Autodesk Fusion 360 part; units mm, degrees
note: some values were not read from the file. Chosen so that the rebuilt part matches the saved one: which face or edge a step refers to.
(part 2 of 3)
sketch "Sketch3" plane through (0, 40, 0) normal (0, 1, 0) x (-1, 0, 0)
  line L0 (-7.2987, -37.3386) -> (-8.9484, -42.0586)
  line L1 (-8.9484, -42.0586) -> (-18.3884, -38.7592)
  line L2 (-18.3884, -38.7592) -> (-16.655, -33.7998)
  line L3 (-16.655, -33.7998) -> (-15.239, -34.2947)
  line L4 (-15.239, -34.2947) -> (-15.0741, -33.8227)
  line L5 (-15.0741, -33.8227) -> (-16.514, -33.2432)
  arc A0 (-16.514, -33.2432) -> (-17.1415, -33.4711) centre (-16.7007, -33.7071) ccw
  line L6 (-17.1415, -33.4711) -> (-19.6803, -38.2133)
  line L7 (-19.6803, -38.2133) -> (-21.5, -37.2391)
  line L8 (-21.5, -37.2391) -> (-18.9559, -32.8326)
  arc A1 (-18.9559, -32.8326) -> (-19.1397, -32.0918) centre (-19.4322, -32.5576) ccw
  line L9 (-19.1397, -32.0918) -> (-20.474, -31.254)
  line L10 (-20.474, -31.254) -> (-20.7904, -31.6411)
  line L11 (-20.7904, -31.6411) -> (-19.6291, -32.5905)
  line L12 (-19.6291, -32.5905) -> (-22.7936, -36.4616)
  line L13 (-22.7936, -36.4616) -> (-30.5359, -30.1325)
  line L14 (-30.5359, -30.1325) -> (-27.2108, -26.0651)
  line L15 (-27.2108, -26.0651) -> (-26.0495, -27.0145)
  line L16 (-26.0495, -27.0145) -> (-25.733, -26.6273)
  line L17 (-25.733, -26.6273) -> (-26.888, -25.5903)
  arc A2 (-26.888, -25.5903) -> (-27.5555, -25.5898) centre (-27.222, -25.9623) ccw
  line L18 (-27.5555, -25.5898) -> (-31.5631, -29.1777)
  line L19 (-31.5631, -29.1777) -> (-32.9399, -27.6399)
  line L20 (-32.9399, -27.6399) -> (-29.0421, -24.3692)
  arc A3 (-29.0421, -24.3692) -> (-28.9615, -23.6103) centre (-29.3957, -23.9479) ccw
  line L21 (-28.9615, -23.6103) -> (-29.9287, -22.3667)
  line L22 (-29.9287, -22.3667) -> (-30.3585, -22.6222)
  line L23 (-30.3585, -22.6222) -> (-29.5919, -23.9115)
  line L24 (-29.5919, -23.9115) -> (-33.8896, -26.4669)
  line L25 (-33.8896, -26.4669) -> (-39.0003, -17.8714)
  line L26 (-39.0003, -17.8714) -> (-34.4846, -15.1865)
  line L27 (-34.4846, -15.1865) -> (-33.718, -16.4758)
  line L28 (-33.718, -16.4758) -> (-33.2882, -16.2203)
  line L29 (-33.2882, -16.2203) -> (-34.0188, -14.8508)
  arc A4 (-34.0188, -14.8508) -> (-34.6459, -14.622) centre (-34.46, -15.0861) ccw
  line L30 (-34.6459, -14.622) -> (-39.639, -16.6229)
  line L31 (-39.639, -16.6229) -> (-40.4068, -14.7069)
  line L32 (-40.4068, -14.7069) -> (-35.6255, -12.9666)
  arc A5 (-35.6255, -12.9666) -> (-35.2901, -12.281) centre (-35.8136, -12.4498) ccw
  line L33 (-35.2901, -12.281) -> (-35.7737, -10.7816)
  line L34 (-35.7737, -10.7816) -> (-36.2649, -10.8747)
  line L35 (-36.2649, -10.8747) -> (-35.9855, -12.3485)
  line L36 (-35.9855, -12.3485) -> (-40.898, -13.2798)
  line L37 (-40.898, -13.2798) -> (-42.7607, -3.4548)
  line L38 (-42.7607, -3.4548) -> (-37.599, -2.4762)
  line L39 (-37.599, -2.4762) -> (-37.3196, -3.95)
  line L40 (-37.3196, -3.95) -> (-36.8284, -3.8568)
  line L41 (-36.8284, -3.8568) -> (-37.0465, -2.3201)
  arc A6 (-37.0465, -2.3201) -> (-37.5576, -1.8906) centre (-37.5415, -2.3903) ccw
  line L42 (-37.5576, -1.8906) -> (-42.9338, -2.063)
  line L43 (-42.9338, -2.063) -> (-43, 0)
  line L44 (-43, 0) -> (-37.9118, 0)
  arc A7 (-37.9118, 0) -> (-37.3622, 0.5296) centre (-37.9118, 0.55) ccw
  line L45 (-37.3622, 0.5296) -> (-37.3038, 2.1039)
  line L46 (-37.3038, 2.1039) -> (-37.7972, 2.1844)
  line L47 (-37.7972, 2.1844) -> (-38.0387, 0.704)
  line L48 (-38.0387, 0.704) -> (-42.9735, 1.509)
  line L49 (-42.9735, 1.509) -> (-41.3635, 11.3786)
  line L50 (-41.3635, 11.3786) -> (-36.1784, 10.5327)
  line L51 (-36.1784, 10.5327) -> (-36.4199, 9.0523)
  line L52 (-36.4199, 9.0523) -> (-35.9265, 8.9718)
  line L53 (-35.9265, 8.9718) -> (-35.6058, 10.4905)
  arc A8 (-35.6058, 10.4905) -> (-35.9392, 11.0689) centre (-36.095, 10.5938) ccw
  line L54 (-35.9392, 11.0689) -> (-36.4082, 11.2228)
  line L55 (-41.0502, 12.7456) -> (-40.4068, 14.7069)
  line L56 (-40.4068, 14.7069) -> (-35.6255, 12.9666)
  arc A9 (-35.6255, 12.9666) -> (-34.9278, 13.2763) centre (-35.4373, 13.4834) ccw
  line L57 (-34.9278, 13.2763) -> (-34.3345, 14.7357)
  line L58 (-34.3345, 14.7357) -> (-34.7707, 14.9801)
  line L59 (-34.7707, 14.9801) -> (-35.5039, 13.6716)
  line L60 (-35.5039, 13.6716) -> (-39.8658, 16.1158)
  line L61 (-39.8658, 16.1158) -> (-34.9773, 24.8395)
  line L62 (-34.9773, 24.8395) -> (-30.3942, 22.2713)
  line L63 (-30.3942, 22.2713) -> (-31.1275, 20.9627)
  line L64 (-31.1275, 20.9627) -> (-30.6913, 20.7183)
  line L65 (-30.6913, 20.7183) -> (-29.8706, 22.0358)
  arc A10 (-29.8706, 22.0358) -> (-29.986, 22.6933) centre (-30.2949, 22.3001) ccw
  line L66 (-29.986, 22.6933) -> (-34.2153, 26.0169)
  line L67 (-34.2153, 26.0169) -> (-32.9399, 27.6399)
  line L68 (-32.9399, 27.6399) -> (-29.0421, 24.3692)
  arc A11 (-29.0421, 24.3692) -> (-28.2807, 24.4217) centre (-28.6886, 24.7906) ccw
  line L69 (-28.2807, 24.4217) -> (-27.2239, 25.5901)
  line L70 (-27.2239, 25.5901) -> (-27.5502, 25.969)
  line L71 (-27.5502, 25.969) -> (-28.6868, 24.9901)
  line L72 (-28.6868, 24.9901) -> (-31.9496, 28.7788)
  line L73 (-31.9496, 28.7788) -> (-24.3723, 35.3044)
  line L74 (-24.3723, 35.3044) -> (-20.944, 31.3236)
  line L75 (-20.944, 31.3236) -> (-22.0806, 30.3448)
  line L76 (-22.0806, 30.3448) -> (-21.7543, 29.9659)
  line L77 (-21.7543, 29.9659) -> (-20.5325, 30.9232)
  arc A12 (-20.5325, 30.9232) -> (-20.4161, 31.5805) centre (-20.8408, 31.3168) ccw
  line L78 (-20.4161, 31.5805) -> (-23.2536, 36.1503)
  line L79 (-23.2536, 36.1503) -> (-21.5, 37.2391)
  line L80 (-21.5, 37.2391) -> (-18.9559, 32.8326)
  arc A13 (-18.9559, 32.8326) -> (-18.2224, 32.6214) centre (-18.4796, 33.1076) ccw
  line L81 (-18.2224, 32.6214) -> (-16.8298, 33.358)
  line L82 (-16.8298, 33.358) -> (-17.0068, 33.8256)
  line L83 (-17.0068, 33.8256) -> (-18.4097, 33.2945)
  line L84 (-18.4097, 33.2945) -> (-20.1799, 37.9707)
  line L85 (-20.1799, 37.9707) -> (-10.8276, 41.5111)
  line L86 (-10.8276, 41.5111) -> (-8.9676, 36.5978)
  line L87 (-8.9676, 36.5978) -> (-10.3705, 36.0667)
  line L88 (-10.3705, 36.0667) -> (-10.1934, 35.5991)
  line L89 (-10.1934, 35.5991) -> (-8.7179, 36.0808)
  arc A14 (-8.7179, 36.0808) -> (-8.3837, 36.6587) centre (-8.873, 36.5561) ccw
  line L90 (-8.3837, 36.6587) -> (-9.4871, 41.9233)
  line L91 (-9.4871, 41.9233) -> (-7.4669, 42.3467)
  line L92 (-7.4669, 42.3467) -> (-6.5833, 37.3358)
  arc A15 (-6.5833, 37.3358) -> (-5.9663, 36.8865) centre (-6.0417, 37.4314) ccw
  line L93 (-5.9663, 36.8865) -> (-4.4057, 37.1024)
  line L94 (-4.4057, 37.1024) -> (-4.4122, 37.6023)
  line L95 (-4.4122, 37.6023) -> (-5.912, 37.5831)
  line L96 (-5.912, 37.5831) -> (-5.9762, 42.5827)
  line L97 (-5.9762, 42.5827) -> (4.023, 42.711)
  line L98 (4.023, 42.711) -> (4.0904, 37.4578)
  line L99 (4.0904, 37.4578) -> (2.5905, 37.4386)
  line L100 (2.5905, 37.4386) -> (2.5969, 36.9386)
  line L101 (2.5969, 36.9386) -> (4.1482, 36.8865)
  arc A16 (4.1482, 36.8865) -> (4.6599, 37.3153) centre (4.165, 37.3863) ccw
  line L102 (4.6599, 37.3153) -> (5.4237, 42.6398)
  line L103 (5.4237, 42.6398) -> (7.4669, 42.3467)
  line L104 (7.4669, 42.3467) -> (6.5833, 37.3358)
  arc A17 (6.5833, 37.3358) -> (7.0094, 36.7026) centre (7.125, 37.2403) ccw
  line L105 (7.0094, 36.7026) -> (8.5497, 36.3717)
  line L106 (8.5497, 36.3717) -> (8.7147, 36.8437)
  line L107 (8.7147, 36.8437) -> (7.2987, 37.3386)
  line L108 (7.2987, 37.3386) -> (8.9484, 42.0586)
  line L109 (8.9484, 42.0586) -> (18.3884, 38.7592)
  line L110 (18.3884, 38.7592) -> (16.655, 33.7998)
  line L111 (16.655, 33.7998) -> (15.239, 34.2947)
  line L112 (15.239, 34.2947) -> (15.0741, 33.8227)
  line L113 (15.0741, 33.8227) -> (16.514, 33.2432)
  arc A18 (16.514, 33.2432) -> (17.1415, 33.4711) centre (16.7007, 33.7071) ccw
  line L114 (17.1415, 33.4711) -> (19.6803, 38.2133)
  line L115 (19.6803, 38.2133) -> (21.5, 37.2391)
  line L116 (21.5, 37.2391) -> (18.9559, 32.8326)
  arc A19 (18.9559, 32.8326) -> (19.1397, 32.0918) centre (19.4322, 32.5576) ccw
  line L117 (19.1397, 32.0918) -> (20.474, 31.254)
  line L118 (20.474, 31.254) -> (20.7904, 31.6411)
  line L119 (20.7904, 31.6411) -> (19.6291, 32.5905)
  line L120 (19.6291, 32.5905) -> (22.7936, 36.4616)
  line L121 (22.7936, 36.4616) -> (30.5359, 30.1325)
  line L122 (30.5359, 30.1325) -> (27.2108, 26.0651)
  line L123 (27.2108, 26.0651) -> (26.0495, 27.0145)
  line L124 (26.0495, 27.0145) -> (25.733, 26.6273)
  line L125 (25.733, 26.6273) -> (26.888, 25.5903)
  arc A20 (26.888, 25.5903) -> (27.5555, 25.5898) centre (27.222, 25.9623) ccw
  line L126 (27.5555, 25.5898) -> (31.5631, 29.1777)
  line L127 (31.5631, 29.1777) -> (32.9399, 27.6399)
  line L128 (32.9399, 27.6399) -> (29.0421, 24.3692)
  arc A21 (29.0421, 24.3692) -> (28.9615, 23.6103) centre (29.3957, 23.9479) ccw
  line L129 (28.9615, 23.6103) -> (29.9287, 22.3667)
  line L130 (29.9287, 22.3667) -> (30.3585, 22.6222)
  line L131 (30.3585, 22.6222) -> (29.5919, 23.9115)
  line L132 (29.5919, 23.9115) -> (33.8896, 26.4669)
  line L133 (33.8896, 26.4669) -> (39.0003, 17.8714)
  line L134 (39.0003, 17.8714) -> (34.4846, 15.1865)
  line L135 (34.4846, 15.1865) -> (33.718, 16.4758)
  line L136 (33.718, 16.4758) -> (33.2882, 16.2203)
  line L137 (33.2882, 16.2203) -> (34.0188, 14.8508)
  arc A22 (34.0188, 14.8508) -> (34.6459, 14.622) centre (34.46, 15.0861) ccw
  line L138 (34.6459, 14.622) -> (39.639, 16.6229)
  line L139 (39.639, 16.6229) -> (40.4068, 14.7069)
  line L140 (40.4068, 14.7069) -> (35.6255, 12.9666)
  arc A23 (35.6255, 12.9666) -> (35.2901, 12.281) centre (35.8136, 12.4498) ccw
  line L141 (35.2901, 12.281) -> (35.7737, 10.7816)
  line L142 (35.7737, 10.7816) -> (36.2649, 10.8747)
  line L143 (36.2649, 10.8747) -> (35.9855, 12.3485)
  line L144 (35.9855, 12.3485) -> (40.898, 13.2798)
  line L145 (40.898, 13.2798) -> (42.7607, 3.4548)
  line L146 (42.7607, 3.4548) -> (37.599, 2.4762)
  line L147 (37.599, 2.4762) -> (37.3196, 3.95)
  line L148 (37.3196, 3.95) -> (36.8284, 3.8568)
  line L149 (36.8284, 3.8568) -> (37.0465, 2.3201)
  arc A24 (37.0465, 2.3201) -> (37.5576, 1.8906) centre (37.5415, 2.3903) ccw
  line L150 (37.5576, 1.8906) -> (42.9338, 2.063)
  line L151 (42.9338, 2.063) -> (43, 0)
  line L152 (43, 0) -> (37.9118, 0)
  arc A25 (37.9118, 0) -> (37.3622, -0.5296) centre (37.9118, -0.55) ccw
  line L153 (37.3622, -0.5296) -> (37.3038, -2.1039)
  line L154 (37.3038, -2.1039) -> (37.7972, -2.1844)
  line L155 (37.7972, -2.1844) -> (38.0387, -0.704)
  line L156 (38.0387, -0.704) -> (42.9735, -1.509)
  line L157 (42.9735, -1.509) -> (41.3635, -11.3786)
  line L158 (41.3635, -11.3786) -> (36.1784, -10.5327)
  line L159 (36.1784, -10.5327) -> (36.4199, -9.0523)
  line L160 (36.4199, -9.0523) -> (35.9265, -8.9718)
  line L161 (35.9265, -8.9718) -> (35.6058, -10.4905)
  arc A26 (35.6058, -10.4905) -> (35.9392, -11.0689) centre (36.095, -10.5938) ccw
  line L162 (35.9392, -11.0689) -> (41.0502, -12.7456)
  line L163 (41.0502, -12.7456) -> (40.4068, -14.7069)
  line L164 (40.4068, -14.7069) -> (35.6255, -12.9666)
  arc A27 (35.6255, -12.9666) -> (34.9278, -13.2763) centre (35.4373, -13.4834) ccw
  line L165 (34.9278, -13.2763) -> (34.3345, -14.7357)
  line L166 (34.3345, -14.7357) -> (34.7707, -14.9801)
  line L167 (34.7707, -14.9801) -> (35.5039, -13.6716)
  line L168 (35.5039, -13.6716) -> (39.8658, -16.1158)
  line L169 (39.8658, -16.1158) -> (34.9773, -24.8395)
  line L170 (34.9773, -24.8395) -> (30.3942, -22.2713)
  line L171 (30.3942, -22.2713) -> (31.1275, -20.9627)
  line L172 (31.1275, -20.9627) -> (30.6913, -20.7183)
  line L173 (30.6913, -20.7183) -> (29.8706, -22.0358)
  arc A28 (29.8706, -22.0358) -> (29.986, -22.6933) centre (30.2949, -22.3001) ccw
  line L174 (29.986, -22.6933) -> (34.2153, -26.0169)
  line L175 (34.2153, -26.0169) -> (32.9399, -27.6399)
  line L176 (32.9399, -27.6399) -> (29.0421, -24.3692)
  arc A29 (29.0421, -24.3692) -> (28.2807, -24.4217) centre (28.6886, -24.7906) ccw
  line L177 (28.2807, -24.4217) -> (27.2239, -25.5901)
  line L178 (27.2239, -25.5901) -> (27.5502, -25.969)
  line L179 (27.5502, -25.969) -> (28.6868, -24.9901)
  line L180 (28.6868, -24.9901) -> (31.9496, -28.7788)
  line L181 (31.9496, -28.7788) -> (24.3723, -35.3044)
  line L182 (24.3723, -35.3044) -> (20.944, -31.3236)
  line L183 (20.944, -31.3236) -> (22.0806, -30.3448)
  line L184 (22.0806, -30.3448) -> (21.7543, -29.9659)
  line L185 (21.7543, -29.9659) -> (20.5325, -30.9232)
  arc A30 (20.5325, -30.9232) -> (20.4161, -31.5805) centre (20.8408, -31.3168) ccw
  line L186 (20.4161, -31.5805) -> (23.2536, -36.1503)
  line L187 (23.2536, -36.1503) -> (21.5, -37.2391)
  line L188 (21.5, -37.2391) -> (18.9559, -32.8326)
  arc A31 (18.9559, -32.8326) -> (18.2224, -32.6214) centre (18.4796, -33.1076) ccw
  line L189 (18.2224, -32.6214) -> (16.8298, -33.358)
  line L190 (16.8298, -33.358) -> (17.0068, -33.8256)
  line L191 (17.0068, -33.8256) -> (18.4097, -33.2945)
  line L192 (18.4097, -33.2945) -> (20.1799, -37.9707)
  line L193 (20.1799, -37.9707) -> (10.8276, -41.5111)
  line L194 (10.8276, -41.5111) -> (8.9676, -36.5978)
  line L195 (8.9676, -36.5978) -> (10.3705, -36.0667)
  line L196 (10.3705, -36.0667) -> (10.1934, -35.5991)
  line L197 (10.1934, -35.5991) -> (8.7179, -36.0808)
  arc A32 (8.7179, -36.0808) -> (8.3837, -36.6587) centre (8.873, -36.5561) ccw
  line L198 (8.3837, -36.6587) -> (9.4871, -41.9233)
  line L199 (9.4871, -41.9233) -> (7.4669, -42.3467)
  line L200 (7.4669, -42.3467) -> (6.5833, -37.3358)
  arc A33 (6.5833, -37.3358) -> (5.9663, -36.8865) centre (6.0417, -37.4314) ccw
  line L201 (5.9663, -36.8865) -> (4.4057, -37.1024)
  line L202 (4.4057, -37.1024) -> (4.4122, -37.6023)
  line L203 (4.4122, -37.6023) -> (5.912, -37.5831)
  line L204 (5.912, -37.5831) -> (5.9762, -42.5827)
  line L205 (5.9762, -42.5827) -> (-4.023, -42.711)
  line L206 (-4.023, -42.711) -> (-4.0904, -37.4578)
  line L207 (-4.0904, -37.4578) -> (-2.5905, -37.4386)
  line L208 (-2.5905, -37.4386) -> (-2.5969, -36.9386)
  line L209 (-2.5969, -36.9386) -> (-4.1482, -36.8865)
  arc A34 (-4.1482, -36.8865) -> (-4.6599, -37.3153) centre (-4.165, -37.3863) ccw
  line L210 (-4.6599, -37.3153) -> (-5.4237, -42.6398)
  line L211 (-5.4237, -42.6398) -> (-7.4669, -42.3467)
  line L212 (-7.4669, -42.3467) -> (-6.5833, -37.3358)
  arc A35 (-6.5833, -37.3358) -> (-7.0094, -36.7026) centre (-7.125, -37.2403) ccw
  line L213 (-7.0094, -36.7026) -> (-8.5497, -36.3717)
  line L214 (-8.5497, -36.3717) -> (-8.7147, -36.8437)
  line L215 (-8.7147, -36.8437) -> (-7.2987, -37.3386)
  circle A36 centre (0, 0) radius 49
  circle A37 centre (0, 0) radius 43
  circle A38 centre (0, 0) radius 46
  line L216 (-36.4082, 11.2228) -> (-41.0502, 12.7456)
  dimension "d51" = 3
  constraint concentric A36 A37
  constraint coincident L180.end A37
extrude "Extrude5" add sketch "Sketch3" along normal blind 5 contours A38
sketch "Sketch4" plane through (0, 0, 0) normal (0, -1, 0) x (1, 0, 0)
  line L0 (8.9484, -42.0586) -> (7.2987, -37.3386)
  line L1 (7.2987, -37.3386) -> (8.7147, -36.8437)
  line L2 (8.7147, -36.8437) -> (8.5497, -36.3717)
  line L3 (8.5497, -36.3717) -> (7.0094, -36.7026)
  arc A0 (7.0094, -36.7026) -> (6.5833, -37.3358) centre (7.125, -37.2403) ccw
  line L4 (6.5833, -37.3358) -> (7.4669, -42.3467)
  line L5 (7.4669, -42.3467) -> (5.4237, -42.6398)
  line L6 (5.4237, -42.6398) -> (4.6599, -37.3153)
  arc A1 (4.6599, -37.3153) -> (4.1482, -36.8865) centre (4.165, -37.3863) ccw
  line L7 (4.1482, -36.8865) -> (2.5969, -36.9386)
  line L8 (2.5969, -36.9386) -> (2.5905, -37.4386)
  line L9 (2.5905, -37.4386) -> (4.0904, -37.4578)
  line L10 (4.0904, -37.4578) -> (4.023, -42.711)
  line L11 (4.023, -42.711) -> (-5.9762, -42.5827)
  line L12 (-5.9762, -42.5827) -> (-5.912, -37.5831)
  line L13 (-5.912, -37.5831) -> (-4.4122, -37.6023)
  line L14 (-4.4122, -37.6023) -> (-4.4057, -37.1024)
  line L15 (-4.4057, -37.1024) -> (-5.9663, -36.8865)
  arc A2 (-5.9663, -36.8865) -> (-6.5833, -37.3358) centre (-6.0417, -37.4314) ccw
  line L16 (-6.5833, -37.3358) -> (-7.4669, -42.3467)
  line L17 (-7.4669, -42.3467) -> (-9.4871, -41.9233)
  line L18 (-9.4871, -41.9233) -> (-8.3837, -36.6587)
  arc A3 (-8.3837, -36.6587) -> (-8.7179, -36.0808) centre (-8.873, -36.5561) ccw
  line L19 (-8.7179, -36.0808) -> (-10.1934, -35.5991)
  line L20 (-10.1934, -35.5991) -> (-10.3705, -36.0667)
  line L21 (-10.3705, -36.0667) -> (-8.9676, -36.5978)
  line L22 (-8.9676, -36.5978) -> (-10.8276, -41.5111)
  line L23 (-10.8276, -41.5111) -> (-20.1799, -37.9707)
  line L24 (-20.1799, -37.9707) -> (-18.4097, -33.2945)
  line L25 (-18.4097, -33.2945) -> (-17.0068, -33.8256)
  line L26 (-17.0068, -33.8256) -> (-16.8298, -33.358)
  line L27 (-16.8298, -33.358) -> (-18.2224, -32.6214)
  arc A4 (-18.2224, -32.6214) -> (-18.9559, -32.8326) centre (-18.4796, -33.1076) ccw
  line L28 (-18.9559, -32.8326) -> (-21.5, -37.2391)
  line L29 (-21.5, -37.2391) -> (-23.2536, -36.1503)
  line L30 (-23.2536, -36.1503) -> (-20.4161, -31.5805)
  arc A5 (-20.4161, -31.5805) -> (-20.5325, -30.9232) centre (-20.8408, -31.3168) ccw
  line L31 (-20.5325, -30.9232) -> (-21.7543, -29.9659)
  line L32 (-21.7543, -29.9659) -> (-22.0806, -30.3448)
  line L33 (-22.0806, -30.3448) -> (-20.944, -31.3236)
  line L34 (-20.944, -31.3236) -> (-24.3723, -35.3044)
  line L35 (-24.3723, -35.3044) -> (-31.9496, -28.7788)
  line L36 (-31.9496, -28.7788) -> (-28.6868, -24.9901)
  line L37 (-28.6868, -24.9901) -> (-27.5502, -25.969)
  line L38 (-27.5502, -25.969) -> (-27.2239, -25.5901)
  line L39 (-27.2239, -25.5901) -> (-28.2807, -24.4217)
  arc A6 (-28.2807, -24.4217) -> (-29.0421, -24.3692) centre (-28.6886, -24.7906) ccw
  line L40 (-29.0421, -24.3692) -> (-32.9399, -27.6399)
  line L41 (-32.9399, -27.6399) -> (-34.2153, -26.0169)
  line L42 (-34.2153, -26.0169) -> (-29.986, -22.6933)
  arc A7 (-29.986, -22.6933) -> (-29.8706, -22.0358) centre (-30.2949, -22.3001) ccw
  line L43 (-29.8706, -22.0358) -> (-30.6913, -20.7183)
  line L44 (-30.6913, -20.7183) -> (-31.1275, -20.9627)
  line L45 (-31.1275, -20.9627) -> (-30.3942, -22.2713)
  line L46 (-30.3942, -22.2713) -> (-34.9773, -24.8395)
  line L47 (-34.9773, -24.8395) -> (-39.8658, -16.1158)
  line L48 (-39.8658, -16.1158) -> (-35.5039, -13.6716)
  line L49 (-35.5039, -13.6716) -> (-34.7707, -14.9801)
  line L50 (-34.7707, -14.9801) -> (-34.3345, -14.7357)
  line L51 (-34.3345, -14.7357) -> (-34.9278, -13.2763)
  arc A8 (-34.9278, -13.2763) -> (-35.6255, -12.9666) centre (-35.4373, -13.4834) ccw
  line L52 (-35.6255, -12.9666) -> (-40.4068, -14.7069)
  line L53 (-40.4068, -14.7069) -> (-41.0502, -12.7456)
  line L54 (-41.0502, -12.7456) -> (-35.9392, -11.0689)
  arc A9 (-35.9392, -11.0689) -> (-35.6058, -10.4905) centre (-36.095, -10.5938) ccw
  line L55 (-35.6058, -10.4905) -> (-35.9265, -8.9718)
  line L56 (-35.9265, -8.9718) -> (-36.4199, -9.0523)
  line L57 (-36.4199, -9.0523) -> (-36.1784, -10.5327)
  line L58 (-36.1784, -10.5327) -> (-41.3635, -11.3786)
  line L59 (-41.3635, -11.3786) -> (-42.9735, -1.509)
  line L60 (-42.9735, -1.509) -> (-38.0387, -0.704)
  line L61 (-38.0387, -0.704) -> (-37.7972, -2.1844)
  line L62 (-37.7972, -2.1844) -> (-37.3038, -2.1039)
  line L63 (-37.3038, -2.1039) -> (-37.3622, -0.5296)
  arc A10 (-37.3622, -0.5296) -> (-37.9118, 0) centre (-37.9118, -0.55) ccw
  line L64 (-37.9118, 0) -> (-43, 0)
  line L65 (-43, 0) -> (-42.9338, 2.063)
  line L66 (-42.9338, 2.063) -> (-37.5576, 1.8906)
  arc A11 (-37.5576, 1.8906) -> (-37.0465, 2.3201) centre (-37.5415, 2.3903) ccw
  line L67 (-37.0465, 2.3201) -> (-36.8284, 3.8568)
  line L68 (-36.8284, 3.8568) -> (-37.3196, 3.95)
  line L69 (-37.3196, 3.95) -> (-37.599, 2.4762)
  line L70 (-37.599, 2.4762) -> (-42.7607, 3.4548)
  line L71 (-42.7607, 3.4548) -> (-40.898, 13.2798)
  line L72 (-40.898, 13.2798) -> (-35.9855, 12.3485)
  line L73 (-35.9855, 12.3485) -> (-36.2649, 10.8747)
  line L74 (-36.2649, 10.8747) -> (-35.7737, 10.7816)
  line L75 (-35.7737, 10.7816) -> (-35.2901, 12.281)
  arc A12 (-35.2901, 12.281) -> (-35.6255, 12.9666) centre (-35.8136, 12.4498) ccw
  line L76 (-35.6255, 12.9666) -> (-40.4068, 14.7069)
  line L77 (-40.4068, 14.7069) -> (-39.639, 16.6229)
  line L78 (-39.639, 16.6229) -> (-34.6459, 14.622)
  arc A13 (-34.6459, 14.622) -> (-34.0188, 14.8508) centre (-34.46, 15.0861) ccw
  line L79 (-34.0188, 14.8508) -> (-33.2882, 16.2203)
  line L80 (-33.2882, 16.2203) -> (-33.718, 16.4758)
  line L81 (-33.718, 16.4758) -> (-34.4846, 15.1865)
  line L82 (-34.4846, 15.1865) -> (-39.0003, 17.8714)
  line L83 (-39.0003, 17.8714) -> (-33.8896, 26.4669)
  line L84 (-33.8896, 26.4669) -> (-29.5919, 23.9115)
  line L85 (-29.5919, 23.9115) -> (-30.3585, 22.6222)
  line L86 (-30.3585, 22.6222) -> (-29.9287, 22.3667)
  line L87 (-29.9287, 22.3667) -> (-28.9615, 23.6103)
  arc A14 (-28.9615, 23.6103) -> (-29.0421, 24.3692) centre (-29.3957, 23.9479) ccw
  line L88 (-29.0421, 24.3692) -> (-32.9399, 27.6399)
  line L89 (-32.9399, 27.6399) -> (-31.5631, 29.1777)
  line L90 (-31.5631, 29.1777) -> (-27.5555, 25.5898)
  arc A15 (-27.5555, 25.5898) -> (-26.888, 25.5903) centre (-27.222, 25.9623) ccw
  line L91 (-26.888, 25.5903) -> (-25.733, 26.6273)
  line L92 (-25.733, 26.6273) -> (-26.0495, 27.0145)
  line L93 (-26.0495, 27.0145) -> (-27.2108, 26.0651)
  line L94 (-27.2108, 26.0651) -> (-30.5359, 30.1325)
  line L95 (-30.5359, 30.1325) -> (-22.7936, 36.4616)
  line L96 (-22.7936, 36.4616) -> (-19.6291, 32.5905)
  line L97 (-19.6291, 32.5905) -> (-20.7904, 31.6411)
  line L98 (-20.7904, 31.6411) -> (-20.474, 31.254)
  line L99 (-20.474, 31.254) -> (-19.1397, 32.0918)
  arc A16 (-19.1397, 32.0918) -> (-18.9559, 32.8326) centre (-19.4322, 32.5576) ccw
  line L100 (-18.9559, 32.8326) -> (-21.5, 37.2391)
  line L101 (-21.5, 37.2391) -> (-19.6803, 38.2133)
  line L102 (-19.6803, 38.2133) -> (-17.1415, 33.4711)
  arc A17 (-17.1415, 33.4711) -> (-16.514, 33.2432) centre (-16.7007, 33.7071) ccw
  line L103 (-16.514, 33.2432) -> (-15.0741, 33.8227)
  line L104 (-15.0741, 33.8227) -> (-15.239, 34.2947)
  line L105 (-15.239, 34.2947) -> (-16.655, 33.7998)
  line L106 (-16.655, 33.7998) -> (-18.3884, 38.7592)
  line L107 (-18.3884, 38.7592) -> (-8.9484, 42.0586)
  line L108 (-8.9484, 42.0586) -> (-7.2987, 37.3386)
  line L109 (-7.2987, 37.3386) -> (-8.7147, 36.8437)
  line L110 (-8.7147, 36.8437) -> (-8.5497, 36.3717)
  line L111 (-8.5497, 36.3717) -> (-7.0094, 36.7026)
  arc A18 (-7.0094, 36.7026) -> (-6.5833, 37.3358) centre (-7.125, 37.2403) ccw
  line L112 (-6.5833, 37.3358) -> (-7.4669, 42.3467)
  line L113 (-7.4669, 42.3467) -> (-5.4237, 42.6398)
  line L114 (-5.4237, 42.6398) -> (-4.6599, 37.3153)
  arc A19 (-4.6599, 37.3153) -> (-4.1482, 36.8865) centre (-4.165, 37.3863) ccw
  line L115 (-4.1482, 36.8865) -> (-2.5969, 36.9386)
  line L116 (-2.5969, 36.9386) -> (-2.5905, 37.4386)
  line L117 (-2.5905, 37.4386) -> (-4.0904, 37.4578)
  line L118 (-4.0904, 37.4578) -> (-4.023, 42.711)
  line L119 (-4.023, 42.711) -> (5.9762, 42.5827)
  line L120 (5.9762, 42.5827) -> (5.912, 37.5831)
  line L121 (5.912, 37.5831) -> (4.4122, 37.6023)
  line L122 (4.4122, 37.6023) -> (4.4057, 37.1024)
  line L123 (4.4057, 37.1024) -> (5.9663, 36.8865)
  arc A20 (5.9663, 36.8865) -> (6.5833, 37.3358) centre (6.0417, 37.4314) ccw
  line L124 (6.5833, 37.3358) -> (7.4669, 42.3467)
  line L125 (7.4669, 42.3467) -> (9.4871, 41.9233)
  line L126 (9.4871, 41.9233) -> (8.3837, 36.6587)
  arc A21 (8.3837, 36.6587) -> (8.7179, 36.0808) centre (8.873, 36.5561) ccw
  line L127 (8.7179, 36.0808) -> (10.1934, 35.5991)
  line L128 (10.1934, 35.5991) -> (10.3705, 36.0667)
  line L129 (10.3705, 36.0667) -> (8.9676, 36.5978)
  line L130 (8.9676, 36.5978) -> (10.8276, 41.5111)
  line L131 (10.8276, 41.5111) -> (20.1799, 37.9707)
  line L132 (20.1799, 37.9707) -> (18.4097, 33.2945)
  line L133 (18.4097, 33.2945) -> (17.0068, 33.8256)
  line L134 (17.0068, 33.8256) -> (16.8298, 33.358)
  line L135 (16.8298, 33.358) -> (18.2224, 32.6214)
  arc A22 (18.2224, 32.6214) -> (18.9559, 32.8326) centre (18.4796, 33.1076) ccw
  line L136 (18.9559, 32.8326) -> (21.5, 37.2391)
  line L137 (21.5, 37.2391) -> (23.2536, 36.1503)
  line L138 (23.2536, 36.1503) -> (20.4161, 31.5805)
  arc A23 (20.4161, 31.5805) -> (20.5325, 30.9232) centre (20.8408, 31.3168) ccw
  line L139 (20.5325, 30.9232) -> (21.7543, 29.9659)
  line L140 (21.7543, 29.9659) -> (22.0806, 30.3448)
  line L141 (22.0806, 30.3448) -> (20.944, 31.3236)
  line L142 (20.944, 31.3236) -> (24.3723, 35.3044)
  line L143 (24.3723, 35.3044) -> (31.9496, 28.7788)
  line L144 (31.9496, 28.7788) -> (28.6868, 24.9901)
  line L145 (28.6868, 24.9901) -> (27.5502, 25.969)
  line L146 (27.5502, 25.969) -> (27.2239, 25.5901)
  line L147 (27.2239, 25.5901) -> (28.2807, 24.4217)
  arc A24 (28.2807, 24.4217) -> (29.0421, 24.3692) centre (28.6886, 24.7906) ccw
  line L148 (29.0421, 24.3692) -> (32.9399, 27.6399)
  line L149 (32.9399, 27.6399) -> (34.2153, 26.0169)
  line L150 (34.2153, 26.0169) -> (29.986, 22.6933)
  arc A25 (29.986, 22.6933) -> (29.8706, 22.0358) centre (30.2949, 22.3001) ccw
  line L151 (29.8706, 22.0358) -> (30.6913, 20.7183)
  line L152 (30.6913, 20.7183) -> (31.1275, 20.9627)
  line L153 (31.1275, 20.9627) -> (30.3942, 22.2713)
  line L154 (30.3942, 22.2713) -> (34.9773, 24.8395)
  line L155 (34.9773, 24.8395) -> (39.8658, 16.1158)
  line L156 (39.8658, 16.1158) -> (35.5039, 13.6716)
  line L157 (35.5039, 13.6716) -> (34.7707, 14.9801)
  line L158 (34.7707, 14.9801) -> (34.3345, 14.7357)
  line L159 (34.3345, 14.7357) -> (34.9278, 13.2763)
  arc A26 (34.9278, 13.2763) -> (35.6255, 12.9666) centre (35.4373, 13.4834) ccw
  line L160 (35.6255, 12.9666) -> (40.4068, 14.7069)
  line L161 (40.4068, 14.7069) -> (41.0502, 12.7456)
  line L162 (41.0502, 12.7456) -> (36.4082, 11.2228)
  arc A27 (35.9392, 11.0689) -> (35.6058, 10.4905) centre (36.095, 10.5938) ccw
  line L163 (35.6058, 10.4905) -> (35.9265, 8.9718)
  line L164 (35.9265, 8.9718) -> (36.4199, 9.0523)
  line L165 (36.4199, 9.0523) -> (36.1784, 10.5327)
  line L166 (36.1784, 10.5327) -> (41.3635, 11.3786)
  line L167 (41.3635, 11.3786) -> (42.9735, 1.509)
  line L168 (42.9735, 1.509) -> (38.0387, 0.704)
  line L169 (38.0387, 0.704) -> (37.7972, 2.1844)
  line L170 (37.7972, 2.1844) -> (37.3038, 2.1039)
  line L171 (37.3038, 2.1039) -> (37.3622, 0.5296)
  arc A28 (37.3622, 0.5296) -> (37.9118, 0) centre (37.9118, 0.55) ccw
  line L172 (37.9118, 0) -> (43, 0)
  line L173 (43, 0) -> (42.9338, -2.063)
  line L174 (42.9338, -2.063) -> (37.5576, -1.8906)
  arc A29 (37.5576, -1.8906) -> (37.0465, -2.3201) centre (37.5415, -2.3903) ccw
  line L175 (37.0465, -2.3201) -> (36.8284, -3.8568)
  line L176 (36.8284, -3.8568) -> (37.3196, -3.95)
  line L177 (37.3196, -3.95) -> (37.599, -2.4762)
  line L178 (37.599, -2.4762) -> (42.7607, -3.4548)
  line L179 (42.7607, -3.4548) -> (40.898, -13.2798)
  line L180 (40.898, -13.2798) -> (35.9855, -12.3485)
  line L181 (35.9855, -12.3485) -> (36.2649, -10.8747)
  line L182 (36.2649, -10.8747) -> (35.7737, -10.7816)
  line L183 (35.7737, -10.7816) -> (35.2901, -12.281)
  arc A30 (35.2901, -12.281) -> (35.6255, -12.9666) centre (35.8136, -12.4498) ccw
  line L184 (35.6255, -12.9666) -> (40.4068, -14.7069)
  line L185 (40.4068, -14.7069) -> (39.639, -16.6229)
  line L186 (39.639, -16.6229) -> (34.6459, -14.622)
  arc A31 (34.6459, -14.622) -> (34.0188, -14.8508) centre (34.46, -15.0861) ccw
  line L187 (34.0188, -14.8508) -> (33.2882, -16.2203)
  line L188 (33.2882, -16.2203) -> (33.718, -16.4758)
  line L189 (33.718, -16.4758) -> (34.4846, -15.1865)
  line L190 (34.4846, -15.1865) -> (39.0003, -17.8714)
  line L191 (39.0003, -17.8714) -> (33.8896, -26.4669)
  line L192 (33.8896, -26.4669) -> (29.5919, -23.9115)
  line L193 (29.5919, -23.9115) -> (30.3585, -22.6222)
  line L194 (30.3585, -22.6222) -> (29.9287, -22.3667)
  line L195 (29.9287, -22.3667) -> (28.9615, -23.6103)
  arc A32 (28.9615, -23.6103) -> (29.0421, -24.3692) centre (29.3957, -23.9479) ccw
  line L196 (29.0421, -24.3692) -> (32.9399, -27.6399)
  line L197 (32.9399, -27.6399) -> (31.5631, -29.1777)
  line L198 (31.5631, -29.1777) -> (27.5555, -25.5898)
  arc A33 (27.5555, -25.5898) -> (26.888, -25.5903) centre (27.222, -25.9623) ccw
  line L199 (26.888, -25.5903) -> (25.733, -26.6273)
  line L200 (25.733, -26.6273) -> (26.0495, -27.0145)
  line L201 (26.0495, -27.0145) -> (27.2108, -26.0651)
  line L202 (27.2108, -26.0651) -> (30.5359, -30.1325)
  line L203 (30.5359, -30.1325) -> (22.7936, -36.4616)
  line L204 (22.7936, -36.4616) -> (19.6291, -32.5905)
  line L205 (19.6291, -32.5905) -> (20.7904, -31.6411)
  line L206 (20.7904, -31.6411) -> (20.474, -31.254)
  line L207 (20.474, -31.254) -> (19.1397, -32.0918)
  arc A34 (19.1397, -32.0918) -> (18.9559, -32.8326) centre (19.4322, -32.5576) ccw
  line L208 (18.9559, -32.8326) -> (21.5, -37.2391)
  line L209 (21.5, -37.2391) -> (19.6803, -38.2133)
  line L210 (19.6803, -38.2133) -> (17.1415, -33.4711)
  arc A35 (17.1415, -33.4711) -> (16.514, -33.2432) centre (16.7007, -33.7071) ccw
  line L211 (16.514, -33.2432) -> (15.0741, -33.8227)
  line L212 (15.0741, -33.8227) -> (15.239, -34.2947)
  line L213 (15.239, -34.2947) -> (16.655, -33.7998)
  line L214 (16.655, -33.7998) -> (18.3884, -38.7592)
  line L215 (18.3884, -38.7592) -> (8.9484, -42.0586)
  circle A36 centre (0, 0) radius 49
  circle A37 centre (0, 0) radius 43
  line L216 (36.4082, 11.2228) -> (35.9392, 11.0689)
  circle A38 centre (0, 0) radius 34.5
  dimension "d54" = -8.5
  constraint concentric A36 A37
  constraint coincident L83.end A37
extrude "Extrude6" add sketch "Sketch4" along normal blind 7 contours L0 L1 L2 L3 A0 L4 A37 | L0 L1 L2 L3 A0 L4 L5 L6 A1 L7 L8 L9 L10 L11 L12 L13 L14 L15 A2 L16 L17 L18 A3 L19 L20 L21 L22 L23 L24 L25 L26 L27 A4 L28 L29 L30 A5 L31 L32 L33 L34 L35 L36 L37 L38 L39 A6 L40 L41 L42 A7 L43 L44 L45 L46 L47 L48 L49 L50 L51 A8 L52 L53 L54 A9 L55 L56 L57 L58 L59 L60 L61 L62 L63 A10 L64 L65 L66 A11 L67 L68 L69 L70 L71 L72 L73 L74 L75 A12 L76 L77 L78 A13 L79 L80 L81 L82 L83 L84 L85 L86 L87 A14 L88 L89 L90 A15 L91 L92 L93 L94 L95 L96 L97 L98 L99 A16 L100 L101 L102 A17 L103 L104 L105 L106 L107 L108 L109 L110 L111 A18 L112 L113 L114 A19 L115 L116 L117 L118 L119 L120 L121 L122 L123 A20 L124 L125 L126 A21 L127 L128 L129 L130 L131 L132 L133 L134 L135 A22 L136 L137 L138 A23 L139 L140 L141 L142 L143 L144 L145 L146 L147 A24 L148 L149 L150 A25 L151 L152 L153 L154 L155 L156 L157 L158 L159 A26 L160 L161 L162 A27 L163 L164 L165 L166 L167 L168 L169 L170 L171 A28 L172 L173 L174 A29 L175 L176 L177 L178 L179 L180 L181 L182 L183 A30 L184 L185 L186 A31 L187 L188 L189 L190 L191 L192 L193 L194 L195 A32 L196 L197 L198 A33 L199 L200 L201 L202 L203 L204 L205 L206 L207 A34 L208 L209 L210 A35 L211 L212 L213 L214 L215 L216 | L209 L210 A35 L211 L212 L213 L214 L215 A37 | L5 L6 A1 L7 L8 L9 L10 L11 A37 | L204 L205 L206 L207 A34 L208 A37 | L12 L13 L14 L15 A2 L16 A37 | L197 L198 A33 L199 L200 L201 L202 L203 A37 | L17 L18 A3 L19 L20 L21 L22 L23 A37 | L192 L193 L194 L195 A32 L196 A37 | L24 L25 L26 L27 A4 L28 A37 | L185 L186 A31 L187 L188 L189 L190 L191 A37 | L29 L30 A5 L31 L32 L33 L34 L35 A37 | L180 L181 L182 L183 A30 L184 A37 | L36 L37 L38 L39 A6 L40 A37 | L173 L174 A29 L175 L176 L177 L178 L179 A37 | L41 L42 A7 L43 L44 L45 L46 L47 A37 | L168 L169 L170 L171 A28 L172 A37 | L48 L49 L50 L51 A8 L52 A37 | L161 L162 A27 L163 L164 L165 L166 L167 A37 L216 | L53 L54 A9 L55 L56 L57 L58 L59 A37 | L156 L157 L158 L159 A26 L160 A37 | L60 L61 L62 L63 A10 L64 A37 | L149 L150 A25 L151 L152 L153 L154 L155 A37 | L65 L66 A11 L67 L68 L69 L70 L71 A37 | L144 L145 L146 L147 A24 L148 A37 | L72 L73 L74 L75 A12 L76 A37 | L137 L138 A23 L139 L140 L141 L142 L143 A37 | L77 L78 A13 L79 L80 L81 L82 L83 A37 | L132 L133 L134 L135 A22 L136 A37 | L84 L85 L86 L87 A14 L88 A37 | L125 L126 A21 L127 L128 L129 L130 L131 A37 | L89 L90 A15 L91 L92 L93 L94 L95 A37 | L120 L121 L122 L123 A20 L124 A37 | L96 L97 L98 L99 A16 L100 A37 | L113 L114 A19 L115 L116 L117 L118 L119 A37 | L101 L102 A17 L103 L104 L105 L106 L107 A37 | L108 L109 L110 L111 A18 L112 A37 | A36
sketch "Sketch6" plane through (0, 0, 0) normal (0, 1, 0) x (-1, 0, 0)
  circle A0 centre (0, 0) radius 34.5
  line L0 (-7.2987, -37.3386) -> (-8.7147, -36.8437)
  line L1 (-8.7147, -36.8437) -> (-8.5497, -36.3717)
  line L2 (-8.5497, -36.3717) -> (-7.0094, -36.7026)
  arc A1 (-6.5833, -37.3358) -> (-7.0094, -36.7026) centre (-7.125, -37.2403) ccw
  line L3 (-6.5833, -37.3358) -> (-7.4669, -42.3467)
  line L4 (-7.4669, -42.3467) -> (-5.4237, -42.6398)
  line L5 (-5.4237, -42.6398) -> (-4.6599, -37.3153)
  arc A2 (-4.1482, -36.8865) -> (-4.6599, -37.3153) centre (-4.165, -37.3863) ccw
  line L6 (-4.1482, -36.8865) -> (-2.5969, -36.9386)
  line L7 (-2.5969, -36.9386) -> (-2.5905, -37.4386)
  line L8 (-2.5905, -37.4386) -> (-4.0904, -37.4578)
  line L9 (-4.0904, -37.4578) -> (-4.023, -42.711)
  line L10 (-4.023, -42.711) -> (5.9762, -42.5827)
  line L11 (5.9762, -42.5827) -> (5.912, -37.5831)
  line L12 (5.912, -37.5831) -> (4.4122, -37.6023)
  line L13 (4.4122, -37.6023) -> (4.4057, -37.1024)
  line L14 (4.4057, -37.1024) -> (5.9663, -36.8865)
  arc A3 (6.5833, -37.3358) -> (5.9663, -36.8865) centre (6.0417, -37.4314) ccw
  line L15 (6.5833, -37.3358) -> (7.4669, -42.3467)
  line L16 (7.4669, -42.3467) -> (9.4871, -41.9233)
  line L17 (9.4871, -41.9233) -> (8.3837, -36.6587)
  arc A4 (8.7179, -36.0808) -> (8.3837, -36.6587) centre (8.873, -36.5561) ccw
  line L18 (8.7179, -36.0808) -> (10.1934, -35.5991)
  line L19 (10.1934, -35.5991) -> (10.3705, -36.0667)
  line L20 (10.3705, -36.0667) -> (8.9676, -36.5978)
  line L21 (8.9676, -36.5978) -> (10.8276, -41.5111)
  line L22 (10.8276, -41.5111) -> (20.1799, -37.9707)
  line L23 (20.1799, -37.9707) -> (18.4097, -33.2945)
  line L24 (18.4097, -33.2945) -> (17.0068, -33.8256)
  line L25 (17.0068, -33.8256) -> (16.8298, -33.358)
  line L26 (16.8298, -33.358) -> (18.2224, -32.6214)
  arc A5 (18.9559, -32.8326) -> (18.2224, -32.6214) centre (18.4796, -33.1076) ccw
  line L27 (18.9559, -32.8326) -> (21.5, -37.2391)
  line L28 (21.5, -37.2391) -> (23.2536, -36.1503)
  line L29 (23.2536, -36.1503) -> (20.4161, -31.5805)
  arc A6 (20.5325, -30.9232) -> (20.4161, -31.5805) centre (20.8408, -31.3168) ccw
  line L30 (20.5325, -30.9232) -> (21.7543, -29.9659)
  line L31 (21.7543, -29.9659) -> (22.0806, -30.3448)
  line L32 (22.0806, -30.3448) -> (20.944, -31.3236)
  line L33 (20.944, -31.3236) -> (24.3723, -35.3044)
  line L34 (24.3723, -35.3044) -> (31.9496, -28.7788)
  line L35 (31.9496, -28.7788) -> (28.6868, -24.9901)
  line L36 (28.6868, -24.9901) -> (27.5502, -25.969)
  line L37 (27.5502, -25.969) -> (27.2239, -25.5901)
  line L38 (27.2239, -25.5901) -> (28.2807, -24.4217)
  arc A7 (29.0421, -24.3692) -> (28.2807, -24.4217) centre (28.6886, -24.7906) ccw
  line L39 (29.0421, -24.3692) -> (32.9399, -27.6399)
  line L40 (32.9399, -27.6399) -> (34.2153, -26.0169)
  line L41 (34.2153, -26.0169) -> (29.986, -22.6933)
  arc A8 (29.8706, -22.0358) -> (29.986, -22.6933) centre (30.2949, -22.3001) ccw
  line L42 (29.8706, -22.0358) -> (30.6913, -20.7183)
  line L43 (30.6913, -20.7183) -> (31.1275, -20.9627)
  line L44 (31.1275, -20.9627) -> (30.3942, -22.2713)
  line L45 (30.3942, -22.2713) -> (34.9773, -24.8395)
  line L46 (34.9773, -24.8395) -> (39.8658, -16.1158)
  line L47 (39.8658, -16.1158) -> (35.5039, -13.6716)
  line L48 (35.5039, -13.6716) -> (34.7707, -14.9801)
  line L49 (34.7707, -14.9801) -> (34.3345, -14.7357)
  line L50 (34.3345, -14.7357) -> (34.9278, -13.2763)
  arc A9 (35.6255, -12.9666) -> (34.9278, -13.2763) centre (35.4373, -13.4834) ccw
  line L51 (35.6255, -12.9666) -> (40.4068, -14.7069)
  line L52 (40.4068, -14.7069) -> (41.0502, -12.7456)
  line L53 (41.0502, -12.7456) -> (35.9392, -11.0689)
  arc A10 (35.6058, -10.4905) -> (35.9392, -11.0689) centre (36.095, -10.5938) ccw
  line L54 (35.6058, -10.4905) -> (35.9265, -8.9718)
  line L55 (35.9265, -8.9718) -> (36.4199, -9.0523)
  line L56 (36.4199, -9.0523) -> (36.1784, -10.5327)
  line L57 (36.1784, -10.5327) -> (41.3635, -11.3786)
  line L58 (41.3635, -11.3786) -> (42.9735, -1.509)
  line L59 (42.9735, -1.509) -> (38.0387, -0.704)
  line L60 (38.0387, -0.704) -> (37.7972, -2.1844)
  line L61 (37.7972, -2.1844) -> (37.3038, -2.1039)
  line L62 (37.3038, -2.1039) -> (37.3622, -0.5296)
  arc A11 (37.9118, 0) -> (37.3622, -0.5296) centre (37.9118, -0.55) ccw
  line L63 (37.9118, 0) -> (43, 0)
  line L64 (43, 0) -> (42.9338, 2.063)
  line L65 (42.9338, 2.063) -> (37.5576, 1.8906)
  arc A12 (37.0465, 2.3201) -> (37.5576, 1.8906) centre (37.5415, 2.3903) ccw
  line L66 (37.0465, 2.3201) -> (36.8284, 3.8568)
  line L67 (36.8284, 3.8568) -> (37.3196, 3.95)
  line L68 (37.3196, 3.95) -> (37.599, 2.4762)
  line L69 (37.599, 2.4762) -> (42.7607, 3.4548)
  line L70 (42.7607, 3.4548) -> (40.898, 13.2798)
  line L71 (40.898, 13.2798) -> (35.9855, 12.3485)
  line L72 (35.9855, 12.3485) -> (36.2649, 10.8747)
  line L73 (36.2649, 10.8747) -> (35.7737, 10.7816)
  line L74 (35.7737, 10.7816) -> (35.2901, 12.281)
  arc A13 (35.6255, 12.9666) -> (35.2901, 12.281) centre (35.8136, 12.4498) ccw
  line L75 (35.6255, 12.9666) -> (40.4068, 14.7069)
  line L76 (40.4068, 14.7069) -> (39.639, 16.6229)
  line L77 (39.639, 16.6229) -> (34.6459, 14.622)
  arc A14 (34.0188, 14.8508) -> (34.6459, 14.622) centre (34.46, 15.0861) ccw
  line L78 (34.0188, 14.8508) -> (33.2882, 16.2203)
  line L79 (33.2882, 16.2203) -> (33.718, 16.4758)
  line L80 (33.718, 16.4758) -> (34.4846, 15.1865)
  line L81 (34.4846, 15.1865) -> (39.0003, 17.8714)
  line L82 (39.0003, 17.8714) -> (33.8896, 26.4669)
  line L83 (33.8896, 26.4669) -> (29.5919, 23.9115)
  line L84 (29.5919, 23.9115) -> (30.3585, 22.6222)
  line L85 (30.3585, 22.6222) -> (29.9287, 22.3667)
  line L86 (29.9287, 22.3667) -> (28.9615, 23.6103)
  arc A15 (29.0421, 24.3692) -> (28.9615, 23.6103) centre (29.3957, 23.9479) ccw
  line L87 (29.0421, 24.3692) -> (32.9399, 27.6399)
  line L88 (32.9399, 27.6399) -> (31.5631, 29.1777)
  line L89 (31.5631, 29.1777) -> (27.5555, 25.5898)
  arc A16 (26.888, 25.5903) -> (27.5555, 25.5898) centre (27.222, 25.9623) ccw
  line L90 (26.888, 25.5903) -> (25.733, 26.6273)
  line L91 (25.733, 26.6273) -> (26.0495, 27.0145)
  line L92 (26.0495, 27.0145) -> (27.2108, 26.0651)
  line L93 (27.2108, 26.0651) -> (30.5359, 30.1325)
  line L94 (30.5359, 30.1325) -> (22.7936, 36.4616)
  line L95 (22.7936, 36.4616) -> (19.6291, 32.5905)
  line L96 (19.6291, 32.5905) -> (20.7904, 31.6411)
  line L97 (20.7904, 31.6411) -> (20.474, 31.254)
  line L98 (20.474, 31.254) -> (19.1397, 32.0918)
  arc A17 (18.9559, 32.8326) -> (19.1397, 32.0918) centre (19.4322, 32.5576) ccw
  line L99 (18.9559, 32.8326) -> (21.5, 37.2391)
  line L100 (21.5, 37.2391) -> (19.6803, 38.2133)
  line L101 (19.6803, 38.2133) -> (17.1415, 33.4711)
  arc A18 (16.514, 33.2432) -> (17.1415, 33.4711) centre (16.7007, 33.7071) ccw
  line L102 (16.514, 33.2432) -> (15.0741, 33.8227)
  line L103 (15.0741, 33.8227) -> (15.239, 34.2947)
  line L104 (15.239, 34.2947) -> (16.655, 33.7998)
  line L105 (16.655, 33.7998) -> (18.3884, 38.7592)
  line L106 (18.3884, 38.7592) -> (8.9484, 42.0586)
  line L107 (8.9484, 42.0586) -> (7.2987, 37.3386)
  line L108 (7.2987, 37.3386) -> (8.7147, 36.8437)
  line L109 (8.7147, 36.8437) -> (8.5497, 36.3717)
  line L110 (8.5497, 36.3717) -> (7.0094, 36.7026)
  arc A19 (6.5833, 37.3358) -> (7.0094, 36.7026) centre (7.125, 37.2403) ccw
  line L111 (6.5833, 37.3358) -> (7.4669, 42.3467)
  line L112 (7.4669, 42.3467) -> (5.4237, 42.6398)
  line L113 (5.4237, 42.6398) -> (4.6599, 37.3153)
  arc A20 (4.1482, 36.8865) -> (4.6599, 37.3153) centre (4.165, 37.3863) ccw
  line L114 (4.1482, 36.8865) -> (2.5969, 36.9386)
  line L115 (2.5969, 36.9386) -> (2.5905, 37.4386)
  line L116 (2.5905, 37.4386) -> (4.0904, 37.4578)
  line L117 (4.0904, 37.4578) -> (4.023, 42.711)
  line L118 (4.023, 42.711) -> (-5.9762, 42.5827)
  line L119 (-5.9762, 42.5827) -> (-5.912, 37.5831)
  line L120 (-5.912, 37.5831) -> (-4.4122, 37.6023)
  line L121 (-4.4122, 37.6023) -> (-4.4057, 37.1024)
  line L122 (-4.4057, 37.1024) -> (-5.9663, 36.8865)
  arc A21 (-6.5833, 37.3358) -> (-5.9663, 36.8865) centre (-6.0417, 37.4314) ccw
  line L123 (-6.5833, 37.3358) -> (-7.4669, 42.3467)
  line L124 (-7.4669, 42.3467) -> (-9.4871, 41.9233)
  line L125 (-9.4871, 41.9233) -> (-8.3837, 36.6587)
  arc A22 (-8.7179, 36.0808) -> (-8.3837, 36.6587) centre (-8.873, 36.5561) ccw
  line L126 (-8.7179, 36.0808) -> (-10.1934, 35.5991)
  line L127 (-10.1934, 35.5991) -> (-10.3705, 36.0667)
  line L128 (-10.3705, 36.0667) -> (-8.9676, 36.5978)
  line L129 (-8.9676, 36.5978) -> (-10.8276, 41.5111)
  line L130 (-10.8276, 41.5111) -> (-20.1799, 37.9707)
  line L131 (-20.1799, 37.9707) -> (-18.4097, 33.2945)
  line L132 (-18.4097, 33.2945) -> (-17.0068, 33.8256)
  line L133 (-17.0068, 33.8256) -> (-16.8298, 33.358)
  line L134 (-16.8298, 33.358) -> (-18.2224, 32.6214)
  arc A23 (-18.9559, 32.8326) -> (-18.2224, 32.6214) centre (-18.4796, 33.1076) ccw
  line L135 (-18.9559, 32.8326) -> (-21.5, 37.2391)
  line L136 (-21.5, 37.2391) -> (-23.2536, 36.1503)
  line L137 (-23.2536, 36.1503) -> (-20.4161, 31.5805)
  arc A24 (-20.5325, 30.9232) -> (-20.4161, 31.5805) centre (-20.8408, 31.3168) ccw
  line L138 (-20.5325, 30.9232) -> (-21.7543, 29.9659)
  line L139 (-21.7543, 29.9659) -> (-22.0806, 30.3448)
  line L140 (-22.0806, 30.3448) -> (-20.944, 31.3236)
  line L141 (-20.944, 31.3236) -> (-24.3723, 35.3044)
  line L142 (-24.3723, 35.3044) -> (-31.9496, 28.7788)
  line L143 (-31.9496, 28.7788) -> (-28.6868, 24.9901)
  line L144 (-28.6868, 24.9901) -> (-27.5502, 25.969)
  line L145 (-27.5502, 25.969) -> (-27.2239, 25.5901)
  line L146 (-27.2239, 25.5901) -> (-28.2807, 24.4217)
  arc A25 (-29.0421, 24.3692) -> (-28.2807, 24.4217) centre (-28.6886, 24.7906) ccw
  line L147 (-29.0421, 24.3692) -> (-32.9399, 27.6399)
  line L148 (-32.9399, 27.6399) -> (-34.2153, 26.0169)
  line L149 (-34.2153, 26.0169) -> (-29.986, 22.6933)
  arc A26 (-29.8706, 22.0358) -> (-29.986, 22.6933) centre (-30.2949, 22.3001) ccw
  line L150 (-29.8706, 22.0358) -> (-30.6913, 20.7183)
  line L151 (-30.6913, 20.7183) -> (-31.1275, 20.9627)
  line L152 (-31.1275, 20.9627) -> (-30.3942, 22.2713)
  line L153 (-30.3942, 22.2713) -> (-34.9773, 24.8395)
  line L154 (-34.9773, 24.8395) -> (-39.8658, 16.1158)
  line L155 (-39.8658, 16.1158) -> (-35.5039, 13.6716)
  line L156 (-35.5039, 13.6716) -> (-34.7707, 14.9801)
  line L157 (-34.7707, 14.9801) -> (-34.3345, 14.7357)
  line L158 (-34.3345, 14.7357) -> (-34.9278, 13.2763)
  arc A27 (-35.6255, 12.9666) -> (-34.9278, 13.2763) centre (-35.4373, 13.4834) ccw
  line L159 (-35.6255, 12.9666) -> (-40.4068, 14.7069)
  line L160 (-40.4068, 14.7069) -> (-41.0502, 12.7456)
  line L161 (-41.0502, 12.7456) -> (-36.4082, 11.2228)
  line L162 (-36.4082, 11.2228) -> (-35.9392, 11.0689)
  arc A28 (-35.6058, 10.4905) -> (-35.9392, 11.0689) centre (-36.095, 10.5938) ccw
  line L163 (-35.6058, 10.4905) -> (-35.9265, 8.9718)
  line L164 (-35.9265, 8.9718) -> (-36.4199, 9.0523)
  line L165 (-36.4199, 9.0523) -> (-36.1784, 10.5327)
  line L166 (-36.1784, 10.5327) -> (-41.3635, 11.3786)
  line L167 (-41.3635, 11.3786) -> (-42.9735, 1.509)
  line L168 (-42.9735, 1.509) -> (-38.0387, 0.704)
  line L169 (-38.0387, 0.704) -> (-37.7972, 2.1844)
  line L170 (-37.7972, 2.1844) -> (-37.3038, 2.1039)
  line L171 (-37.3038, 2.1039) -> (-37.3622, 0.5296)
  arc A29 (-37.9118, 0) -> (-37.3622, 0.5296) centre (-37.9118, 0.55) ccw
  line L172 (-37.9118, 0) -> (-43, 0)
  line L173 (-43, 0) -> (-42.9338, -2.063)
  line L174 (-42.9338, -2.063) -> (-37.5576, -1.8906)
  arc A30 (-37.0465, -2.3201) -> (-37.5576, -1.8906) centre (-37.5415, -2.3903) ccw
  line L175 (-37.0465, -2.3201) -> (-36.8284, -3.8568)
  line L176 (-36.8284, -3.8568) -> (-37.3196, -3.95)
  line L177 (-37.3196, -3.95) -> (-37.599, -2.4762)
  line L178 (-37.599, -2.4762) -> (-42.7607, -3.4548)
  line L179 (-42.7607, -3.4548) -> (-40.898, -13.2798)
  line L180 (-40.898, -13.2798) -> (-35.9855, -12.3485)
  line L181 (-35.9855, -12.3485) -> (-36.2649, -10.8747)
  line L182 (-36.2649, -10.8747) -> (-35.7737, -10.7816)
  line L183 (-35.7737, -10.7816) -> (-35.2901, -12.281)
  arc A31 (-35.6255, -12.9666) -> (-35.2901, -12.281) centre (-35.8136, -12.4498) ccw
  line L184 (-35.6255, -12.9666) -> (-40.4068, -14.7069)
  line L185 (-40.4068, -14.7069) -> (-39.639, -16.6229)
  line L186 (-39.639, -16.6229) -> (-34.6459, -14.622)
  arc A32 (-34.0188, -14.8508) -> (-34.6459, -14.622) centre (-34.46, -15.0861) ccw
  line L187 (-34.0188, -14.8508) -> (-33.2882, -16.2203)
  line L188 (-33.2882, -16.2203) -> (-33.718, -16.4758)
  line L189 (-33.718, -16.4758) -> (-34.4846, -15.1865)
  line L190 (-34.4846, -15.1865) -> (-39.0003, -17.8714)
  line L191 (-39.0003, -17.8714) -> (-33.8896, -26.4669)
  line L192 (-33.8896, -26.4669) -> (-29.5919, -23.9115)
  line L193 (-29.5919, -23.9115) -> (-30.3585, -22.6222)
  line L194 (-30.3585, -22.6222) -> (-29.9287, -22.3667)
  line L195 (-29.9287, -22.3667) -> (-28.9615, -23.6103)
  arc A33 (-29.0421, -24.3692) -> (-28.9615, -23.6103) centre (-29.3957, -23.9479) ccw
  line L196 (-29.0421, -24.3692) -> (-32.9399, -27.6399)
  line L197 (-32.9399, -27.6399) -> (-31.5631, -29.1777)
  line L198 (-31.5631, -29.1777) -> (-27.5555, -25.5898)
  arc A34 (-26.888, -25.5903) -> (-27.5555, -25.5898) centre (-27.222, -25.9623) ccw
  line L199 (-26.888, -25.5903) -> (-25.733, -26.6273)
  line L200 (-25.733, -26.6273) -> (-26.0495, -27.0145)
  line L201 (-26.0495, -27.0145) -> (-27.2108, -26.0651)
  line L202 (-27.2108, -26.0651) -> (-30.5359, -30.1325)
  line L203 (-30.5359, -30.1325) -> (-22.7936, -36.4616)
  line L204 (-22.7936, -36.4616) -> (-19.6291, -32.5905)
  line L205 (-19.6291, -32.5905) -> (-20.7904, -31.6411)
  line L206 (-20.7904, -31.6411) -> (-20.474, -31.254)
  line L207 (-20.474, -31.254) -> (-19.1397, -32.0918)
  arc A35 (-18.9559, -32.8326) -> (-19.1397, -32.0918) centre (-19.4322, -32.5576) ccw
  line L208 (-18.9559, -32.8326) -> (-21.5, -37.2391)
  line L209 (-21.5, -37.2391) -> (-19.6803, -38.2133)
  line L210 (-19.6803, -38.2133) -> (-17.1415, -33.4711)
  arc A36 (-16.514, -33.2432) -> (-17.1415, -33.4711) centre (-16.7007, -33.7071) ccw
  line L211 (-16.514, -33.2432) -> (-15.0741, -33.8227)
  line L212 (-15.0741, -33.8227) -> (-15.239, -34.2947)
  line L213 (-15.239, -34.2947) -> (-16.655, -33.7998)
  line L214 (-16.655, -33.7998) -> (-18.3884, -38.7592)
  line L215 (-18.3884, -38.7592) -> (-8.9484, -42.0586)
  line L216 (-8.9484, -42.0586) -> (-7.2987, -37.3386)
  circle A37 centre (0, 0) radius 37.0298
  constraint coincident A0.centre A37.centre
  constraint coincident L30.end A37
extrude "Extrude7" cut sketch "Sketch6" against normal blind 4.5 contours A37
chamfer "Chamfer1" distance 2.5 angle 45 1 edges at (-32.1653, -4.5, 12.4757)